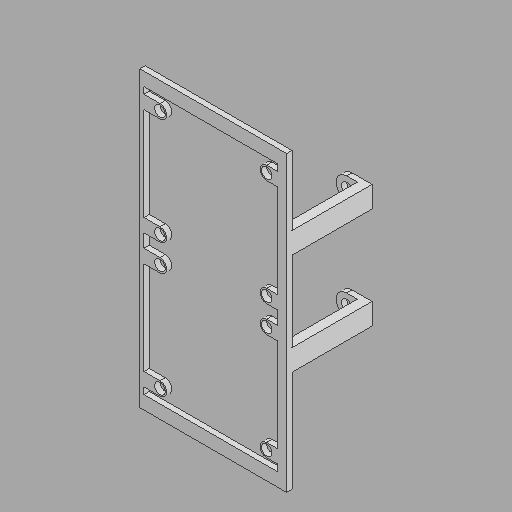
# Autodesk Inventor part: MTN_PLATE_RETROFIT
Saved by Autodesk Inventor 2025.2 (Build 292293000, 293)
## iProperties
Created: 2026-08-10
Part Number: MTN_PLATE_RETROFIT
Material: Generic
Document SubType Name: Modeling
Designer: Ben
Density: 1 g/cm^3
Appearance: Default
Author: Ben
Autodesk Inventor part; units mm, degrees
ref_plane "YZ Plane" through (0, 0, 0) normal (1, 0, 0) x (0, 1, 0)
ref_plane "XZ Plane" through (0, 0, 0) normal (0, 1, 0) x (-1, 0, 0)
ref_plane "XY Plane" through (0, 0, 0) normal (0, 0, 1) x (1, 0, 0)
sketch "Sketch1" plane through (0, 0, 0) normal (0, 0, 1) x (1, 0, 0)
  line L0 (-27.5, -55) -> (27.5, -55)
  line L1 (27.5, -55) -> (27.5, 55)
  line L2 (27.5, 55) -> (-27.5, 55)
  line L3 (-27.5, 55) -> (-27.5, -55)
  line L4 (-27.5, -55) -> (27.5, 55) construction
  line L5 (27.5, -55) -> (-27.5, 55) construction
  line L6 (0, -77) -> (0, 77) projected
  line L7 (-38.5, 0) -> (38.5, 0) projected
  circle A0 centre (-20, 45) radius 2
  circle A1 centre (-20, 5) radius 2
  circle A2 centre (20, 45) radius 2
  circle A3 centre (20, 5) radius 2
  circle A4 centre (-20, -5) radius 2
  circle A5 centre (-20, -45) radius 2
  circle A6 centre (20, -45) radius 2
  circle A7 centre (20, -5) radius 2
  arc A8 (-20, 42.5) -> (-20, 47.5) centre (-20, 45) ccw
  arc A9 (20, 47.5) -> (20, 42.5) centre (20, 45) ccw
  arc A10 (-20, 2.5) -> (-20, 7.5) centre (-20, 5) ccw
  arc A11 (20, 7.5) -> (20, 2.5) centre (20, 5) ccw
  arc A12 (-20, -7.5) -> (-20, -2.5) centre (-20, -5) ccw
  arc A13 (20, -2.5) -> (20, -7.5) centre (20, -5) ccw
  arc A14 (-20, -47.5) -> (-20, -42.5) centre (-20, -45) ccw
  arc A15 (20, -42.5) -> (20, -47.5) centre (20, -45) ccw
  line L8 (-26, -50) -> (24, -50)
  line L9 (24, -50) -> (24, 50)
  line L10 (24, 50) -> (-26, 50)
  line L11 (-26, 50) -> (-26, -50)
  line L12 (-20, 47.5) -> (-26, 47.5)
  line L13 (-20, 42.5) -> (-26, 42.5)
  line L14 (20, 47.5) -> (24, 47.5)
  line L15 (20, 42.5) -> (24, 42.5)
  line L16 (20, 7.5) -> (24, 7.5)
  line L17 (20, 2.5) -> (24, 2.5)
  line L18 (20, -2.5) -> (24, -2.5)
  line L19 (20, -7.5) -> (24, -7.5)
  line L20 (20, -42.5) -> (24, -42.5)
  line L21 (-20, 7.5) -> (-26, 7.5)
  line L22 (-20, 2.5) -> (-26, 2.5)
  line L23 (-20, -2.5) -> (-26, -2.5)
  line L24 (-20, -7.5) -> (-26, -7.5)
  line L25 (-20, -42.5) -> (-26, -42.5)
  line L26 (-20, -47.5) -> (-26, -47.5)
  line L27 (20, -47.5) -> (24, -47.5)
  point P0 (0, 0)
  point P1 (-17.5, 45)
  dimension "d0" = 55
  dimension "d1" = 110
  dimension "d5" = 40
  dimension "d6" = 40
  dimension "d7" = 4
  dimension "d8" = 90
  dimension "d9" = 2.5
  dimension "d10" = 5
  dimension "d12" = 6
  dimension "d13" = 4
  constraints: 48 end point, 17 point on circle, 17 vertical alignment, 16 centre point, 15 horizontal, 8 coincident, 5 parallel, 4 equal radius, 2 midpoint, 2 point on line, 1 perpendicular, 33 other
  measures "d0" distance of L1.end L2.end
  measures "d1" distance of L0.end L1.end
  measures "d5" distance of A1.centre A0.centre
  measures "d6" distance of A2.centre A0.centre
  measures "d7" diameter of A2
  measures "d8" distance of A6.centre A2.centre
  measures "d9" distance of point (-17.5, 45) A8.centre
  measures "d10" distance between parallel lines of L10 L2
extrude "Extrusion1" add sketch "Sketch1" along normal blind 2 contours L3 L7 L11 L8 L6 L0 | L6 L8 L9 L7 L1 L0 | L3 L2 L6 L10 L11 L7 | L7 L9 L10 L6 L2 L1 | L11 L21 A10 L22 | L23 A12 L24 L11 | L11 L25 A14 L26 | L27 A15 L20 L9 | L9 L19 A13 L18 | L17 A11 L16 L9 | L11 L12 A8 L13 | L9 L15 A9 L14
sketch "Sketch3" plane through (0, 0, 0) normal (0, 0, -1) x (-1, 0, 0)
  line L0 (-27.5, 55) -> (27.5, 55) projected
  line L1 (-16, 55) -> (-24, 55)
  line L2 (-27.5, 55) -> (27.5, 55) projected
  line L3 (-27.5, -55) -> (-27.5, 55) projected
  line L4 (27.5, -55) -> (-27.5, -55) projected
  line L5 (27.5, 55) -> (27.5, -55) projected
  circle A0 centre (-20, -5) radius 2 projected
  circle A1 centre (-20, 45) radius 2 projected
  circle A2 centre (20, 45) radius 2 projected
  circle A3 centre (-20, 5) radius 2 projected
  circle A4 centre (20, -5) radius 2 projected
  circle A5 centre (-20, -45) radius 2 projected
  circle A6 centre (20, -45) radius 2 projected
  circle A7 centre (20, 5) radius 2 projected
  line L6 (-24, 2.5) -> (-24, -2.5) projected
  line L7 (-20, 2.5) -> (-24, 2.5) projected
  arc A8 (-20, 2.5) -> (-20, 7.5) centre (-20, 5) ccw projected
  line L8 (-24, 7.5) -> (-20, 7.5) projected
  line L9 (-24, 42.5) -> (-24, 7.5) projected
  line L10 (-20, 42.5) -> (-24, 42.5) projected
  arc A9 (-20, 42.5) -> (-20, 47.5) centre (-20, 45) ccw projected
  line L11 (-24, 47.5) -> (-20, 47.5) projected
  line L12 (-24, 50) -> (-24, 47.5) projected
  line L13 (26, 50) -> (-24, 50) projected
  line L14 (26, 47.5) -> (26, 50) projected
  line L15 (20, 47.5) -> (26, 47.5) projected
  arc A10 (20, 47.5) -> (20, 42.5) centre (20, 45) ccw projected
  line L16 (26, 42.5) -> (20, 42.5) projected
  line L17 (26, 7.5) -> (26, 42.5) projected
  line L18 (20, 7.5) -> (26, 7.5) projected
  arc A11 (20, 7.5) -> (20, 2.5) centre (20, 5) ccw projected
  line L19 (26, 2.5) -> (20, 2.5) projected
  line L20 (26, -2.5) -> (26, 2.5) projected
  line L21 (20, -2.5) -> (26, -2.5) projected
  arc A12 (20, -2.5) -> (20, -7.5) centre (20, -5) ccw projected
  line L22 (26, -7.5) -> (20, -7.5) projected
  line L23 (26, -42.5) -> (26, -7.5) projected
  line L24 (20, -42.5) -> (26, -42.5) projected
  arc A13 (20, -42.5) -> (20, -47.5) centre (20, -45) ccw projected
  line L25 (26, -47.5) -> (20, -47.5) projected
  line L26 (26, -50) -> (26, -47.5) projected
  line L27 (-24, -50) -> (26, -50) projected
  line L28 (-24, -47.5) -> (-24, -50) projected
  line L29 (-20, -47.5) -> (-24, -47.5) projected
  arc A14 (-20, -47.5) -> (-20, -42.5) centre (-20, -45) ccw projected
  line L30 (-24, -42.5) -> (-20, -42.5) projected
  line L31 (-24, -7.5) -> (-24, -42.5) projected
  line L32 (-20, -7.5) -> (-24, -7.5) projected
  arc A15 (-20, -7.5) -> (-20, -2.5) centre (-20, -5) ccw projected
  line L33 (-24, -2.5) -> (-20, -2.5) projected
  line L34 (14, 50) -> (22, 50)
  line L35 (22, 55) -> (14, 55)
  line L36 (-27.5, -17) -> (-24, -17)
  line L37 (-24, -17) -> (-24, -9)
  line L38 (-24, -9) -> (-27.5, -9)
  line L39 (-27.5, -9) -> (-27.5, -17)
  line L40 (-27.5, -17) -> (-24, -9) construction
  line L41 (-24, -17) -> (-27.5, -9) construction
  line L42 (-24, 29) -> (-27.5, 29)
  line L43 (-27.5, 29) -> (-27.5, 21)
  line L44 (-27.5, 21) -> (-24, 21)
  line L45 (-24, 21) -> (-24, 29)
  line L46 (-24, 29) -> (-27.5, 21) construction
  line L47 (-27.5, 29) -> (-24, 21) construction
  point P0 (0, 0)
  point P1 (-25.75, -13)
  point P2 (-27.5, -17)
  point P3 (-24, 10.5)
  point P4 (-25.75, 25)
  dimension "d22" = 8
  dimension "d40" = 38
  dimension "d41" = 25
  constraints: 30 end point, 5 parallel, 4 midpoint, 3 horizontal, 3 point on line, 2 equal length, 2 perpendicular, 1 vertical alignment
  measures "d22" distance of L38.end L36.start
  measures "d40" distance of point (-25.75, 25) point (-25.75, -13)
  measures "d41" distance from line of L13 point (-25.75, 25)
extrude "Extrusion3" add sketch "Sketch3" along normal blind 28 contours L42 L9 L44 L3 | L38 L31 L36 L3
sketch "Sketch5" plane through (0, 0, -28) normal (0, 0, -1) x (-1, 0, 0)
  line L0 (-27.5, -9) -> (-27.5, -17) projected
  line L1 (-24, 21) -> (-24, 29) projected
  circle A0 centre (-20, -13) radius 2
  line L2 (-27.5, -9) -> (-27.5, -17) projected
  arc A1 (-20, -17) -> (-20, -9) centre (-20, -13) ccw
  line L3 (-20, -17) -> (-24, -17)
  line L4 (-24, -9) -> (-20, -9)
  line L5 (-24, -17) -> (-24, -9) projected
  line L6 (-24, 29) -> (-27.5, 29) projected
  line L7 (-27.5, 29) -> (-27.5, 21) projected
  line L8 (-27.5, 21) -> (-24, 21) projected
  line L9 (-27.5, -17) -> (-24, -17) projected
  line L10 (-24, -9) -> (-27.5, -9) projected
  circle A2 centre (-20, 25) radius 2
  arc A3 (-20, 21) -> (-20, 29) centre (-20, 25) ccw
  line L11 (-20, 21) -> (-24, 21)
  line L12 (-24, 29) -> (-27.5, 29) projected
  line L13 (-24, 29) -> (-20, 29)
  point P0 (0, 0)
  point P1 (-27.5, -13)
  point P2 (-27.5, -13)
  point P3 (-16, -13)
  point P4 (-24, 13)
  point P5 (-24, -17)
  point P6 (-24, -9)
  point P7 (-24, 25)
  point P8 (-16, 25)
  dimension "d36" = 4
  dimension "d37" = 8
  constraints: 8 end point, 6 point on circle, 6 vertical alignment, 5 horizontal alignment, 4 centre point, 3 midpoint, 3 parallel, 2 coincident, 1 equal radius, 1 horizontal
  measures "d36" diameter of A0
  measures "d37" distance from line of L1 point (-16, -13)
extrude "Extrusion5" add sketch "Sketch5" along normal blind 2
body "Solid1"
